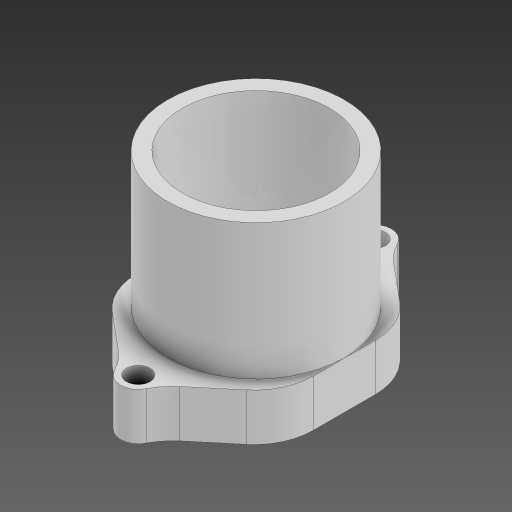
# Autodesk Inventor part: conder
Saved by Autodesk Inventor 2023 (Build 270158000, 158)
## iProperties
Created: 2025-09-15
Part Number: conder
Material: Типовые
Document SubType Name: Modeling
Designer: daa
Density: 1 g/cm^3
Appearance: По умолчанию
Author: daa
Autodesk Inventor part; units mm, degrees
ref_plane "YZ Plane" through (0, 0, 0) normal (1, 0, 0) x (0, 1, 0)
ref_plane "XZ Plane" through (0, 0, 0) normal (0, 1, 0) x (-1, 0, 0)
ref_plane "XY Plane" through (0, 0, 0) normal (0, 0, 1) x (1, 0, 0)
sketch "Эскиз1" plane through (0, 0, 0) normal (0, 1, 0) x (-1, 0, 0)
  circle A0 centre (0, 0) radius 12.5
  circle A1 centre (0, 0) radius 15
  dimension "d0" = 25
  dimension "d1" = 30
  constraints: 2 centre point, 2 coincident
  measures "d0" diameter of A0
  measures "d1" diameter of A1
extrude "Выдавливание1" add sketch "Эскиз1" along normal blind 31
sketch "Эскиз2" plane through (0, 0, 0) normal (0, -1, 0) x (1, 0, 0)
  line L0 (0, 20) -> (0, -20)
  circle A0 centre (0, 20) radius 2
  circle A1 centre (0, -20) radius 2
  circle A2 centre (0, 20) radius 3
  circle A3 centre (0, -20) radius 3
  line L1 (15, 10) -> (15, -10)
  circle A4 centre (0, 0) radius 15 projected
  line L2 (-15, 10) -> (-15, -10)
  line L3 (3, 20) -> (15, 10)
  line L4 (15, -10) -> (3, -20)
  line L5 (-15, -10) -> (-3, -20)
  line L6 (-3, 20) -> (-15, 10)
  point P0 (15, 0)
  point P1 (-15, 0)
  dimension "d4" = 40
  dimension "d5" = 4
  dimension "d6" = 4
  dimension "d7" = 6
  dimension "d8" = 6
  dimension "d9" = 20
  dimension "d10" = 20
  dimension "d11" = 10
  dimension "d12" = 10
  constraints: 14 end point, 5 coincident, 4 centre point, 4 point on circle, 3 vertical, 2 tangent, 1 midpoint, 1 parallel
  measures "d4" distance of L0.start L0.end
  measures "d5" diameter of A0
  measures "d6" diameter of A1
  measures "d7" diameter of A2
  measures "d8" diameter of A3
  measures "d9" distance of L1.start L1.end
  measures "d10" distance of L2.start L2.end
  measures "d11" vertical distance of L1.end point (0, 0)
  measures "d12" vertical distance of point (0, 0) L2.start
extrude "Выдавливание2" add sketch "Эскиз2" against normal blind 8 contours A2 | A2 L3 L1 A4 L0 | L0 A4 L2 L6 A2 | A4 L1 L4 A3 L0 | L0 A3 L5 L2 A4 | A3
fillet "Сопряжение1" radius 10 4 edges at (-15, 4, 10) (-15, 4, -10) (15, 4, 10) (15, 4, -10)
fillet "Сопряжение2" radius 10 4 edges at (3, 4, 20) (-3, 4, 20) (3, 4, -20) (-3, 4, -20)
